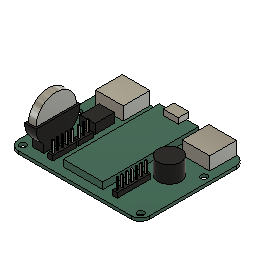
Main_PCB (Autodesk Fusion 360 design; units mm, degrees)
Autodesk Fusion 360 part; units mm, degrees
note: some values were not read from the file. Set by a fixed rule: which sketch regions a step uses.
(part 1 of 3)
sketch "Sketch1" plane through (0, 0, 0) normal (0, 1, 0) x (1, 0, 0)
  line L0 (20.2962, -41.7031) -> (20.1819, -41.6079)
  line L1 (20.1819, -41.6079) -> (20.0105, -41.6079)
  line L2 (20.0105, -41.6079) -> (19.839, -41.7031)
  line L3 (19.839, -41.7031) -> (19.7247, -41.8936)
  line L4 (19.7247, -41.8936) -> (19.6676, -42.0841)
  line L5 (19.6676, -42.0841) -> (19.6105, -42.465)
  line L6 (19.6105, -42.465) -> (19.6105, -42.7507)
  line L7 (19.6105, -42.7507) -> (19.6676, -43.1317)
  line L8 (19.6676, -43.1317) -> (19.7247, -43.3222)
  line L9 (19.7247, -43.3222) -> (19.839, -43.5127)
  line L10 (19.839, -43.5127) -> (20.0105, -43.6079)
  line L11 (20.0105, -43.6079) -> (20.1247, -43.6079)
  line L12 (20.1247, -43.6079) -> (20.2962, -43.5127)
  line L13 (20.2962, -43.5127) -> (20.3533, -43.4174)
  line L14 (20.3533, -43.4174) -> (20.3533, -42.7507)
  line L15 (20.3533, -42.7507) -> (20.1247, -42.7507)
  line L16 (20.8676, -43.6079) -> (20.8676, -41.6079)
  line L17 (20.8676, -41.6079) -> (21.5533, -43.6079)
  line L18 (21.5533, -43.6079) -> (21.5533, -41.6079)
  line L19 (22.1247, -43.6079) -> (22.1247, -41.6079)
  line L20 (22.1247, -41.6079) -> (22.4105, -41.6079)
  line L21 (22.4105, -41.6079) -> (22.5819, -41.7031)
  line L22 (22.5819, -41.7031) -> (22.6962, -41.8936)
  line L23 (22.6962, -41.8936) -> (22.7533, -42.0841)
  line L24 (22.7533, -42.0841) -> (22.8105, -42.465)
  line L25 (22.8105, -42.465) -> (22.8105, -42.7507)
  line L26 (22.8105, -42.7507) -> (22.7533, -43.1317)
  line L27 (22.7533, -43.1317) -> (22.6962, -43.3222)
  line L28 (22.6962, -43.3222) -> (22.5819, -43.5127)
  line L29 (22.5819, -43.5127) -> (22.4105, -43.6079)
  line L30 (22.4105, -43.6079) -> (22.1247, -43.6079)
  line L31 (66.9917, -47.6054) -> (67.0393, -47.4625)
  line L32 (67.0393, -47.4625) -> (67.0393, -47.2244)
  line L33 (67.0393, -47.2244) -> (66.9917, -47.1292)
  line L34 (66.9917, -47.1292) -> (66.9441, -47.0816)
  line L35 (66.9441, -47.0816) -> (66.8489, -47.034)
  line L36 (66.8489, -47.034) -> (66.7536, -47.034)
  line L37 (66.7536, -47.034) -> (66.6584, -47.0816)
  line L38 (66.6584, -47.0816) -> (66.6108, -47.1292)
  line L39 (66.6108, -47.1292) -> (66.5632, -47.2244)
  line L40 (66.5632, -47.2244) -> (66.5155, -47.4149)
  line L41 (66.5155, -47.4149) -> (66.4679, -47.5102)
  line L42 (66.4679, -47.5102) -> (66.4203, -47.5578)
  line L43 (66.4203, -47.5578) -> (66.3251, -47.6054)
  line L44 (66.3251, -47.6054) -> (66.2298, -47.6054)
  line L45 (66.2298, -47.6054) -> (66.1346, -47.5578)
  line L46 (66.1346, -47.5578) -> (66.087, -47.5102)
  line L47 (66.087, -47.5102) -> (66.0393, -47.4149)
  line L48 (66.0393, -47.4149) -> (66.0393, -47.1768)
  line L49 (66.0393, -47.1768) -> (66.087, -47.034)
  line L50 (66.3727, -46.1768) -> (67.0393, -46.1768)
  line L51 (66.3727, -46.6054) -> (66.8965, -46.6054)
  line L52 (66.8965, -46.6054) -> (66.9917, -46.5578)
  line L53 (66.9917, -46.5578) -> (67.0393, -46.4625)
  line L54 (67.0393, -46.4625) -> (67.0393, -46.3197)
  line L55 (67.0393, -46.3197) -> (66.9917, -46.2244)
  line L56 (66.9917, -46.2244) -> (66.9441, -46.1768)
  line L57 (66.3727, -45.7006) -> (67.0393, -45.7006)
  line L58 (66.4679, -45.7006) -> (66.4203, -45.653)
  line L59 (66.4203, -45.653) -> (66.3727, -45.5578)
  line L60 (66.3727, -45.5578) -> (66.3727, -45.4149)
  line L61 (66.3727, -45.4149) -> (66.4203, -45.3197)
  line L62 (66.4203, -45.3197) -> (66.5155, -45.2721)
  line L63 (66.5155, -45.2721) -> (67.0393, -45.2721)
  line L64 (67.0393, -44.7959) -> (66.3727, -44.7959)
  line L65 (66.5632, -44.7959) -> (66.4679, -44.7482)
  line L66 (66.4679, -44.7482) -> (66.4203, -44.7006)
  line L67 (66.4203, -44.7006) -> (66.3727, -44.6054)
  line L68 (66.3727, -44.6054) -> (66.3727, -44.5102)
  line L69 (67.0393, -44.1768) -> (66.3727, -44.1768)
  line L70 (66.0393, -44.1768) -> (66.087, -44.2244)
  line L71 (66.087, -44.2244) -> (66.1346, -44.1768)
  line L72 (66.1346, -44.1768) -> (66.087, -44.1292)
  line L73 (66.087, -44.1292) -> (66.0393, -44.1768)
  line L74 (66.0393, -44.1768) -> (66.1346, -44.1768)
  line L75 (66.9917, -43.7482) -> (67.0393, -43.653)
  line L76 (67.0393, -43.653) -> (67.0393, -43.4625)
  line L77 (67.0393, -43.4625) -> (66.9917, -43.3673)
  line L78 (66.9917, -43.3673) -> (66.8965, -43.3197)
  line L79 (66.8965, -43.3197) -> (66.8489, -43.3197)
  line L80 (66.8489, -43.3197) -> (66.7536, -43.3673)
  line L81 (66.7536, -43.3673) -> (66.706, -43.4625)
  line L82 (66.706, -43.4625) -> (66.706, -43.6054)
  line L83 (66.706, -43.6054) -> (66.6584, -43.7006)
  line L84 (66.6584, -43.7006) -> (66.5632, -43.7482)
  line L85 (66.5632, -43.7482) -> (66.5155, -43.7482)
  line L86 (66.5155, -43.7482) -> (66.4203, -43.7006)
  line L87 (66.4203, -43.7006) -> (66.3727, -43.6054)
  line L88 (66.3727, -43.6054) -> (66.3727, -43.4625)
  line L89 (66.3727, -43.4625) -> (66.4203, -43.3673)
  line L90 (66.9917, -42.5102) -> (67.0393, -42.6054)
  line L91 (67.0393, -42.6054) -> (67.0393, -42.7959)
  line L92 (67.0393, -42.7959) -> (66.9917, -42.8911)
  line L93 (66.9917, -42.8911) -> (66.8965, -42.9387)
  line L94 (66.8965, -42.9387) -> (66.5155, -42.9387)
  line L95 (66.5155, -42.9387) -> (66.4203, -42.8911)
  line L96 (66.4203, -42.8911) -> (66.3727, -42.7959)
  line L97 (66.3727, -42.7959) -> (66.3727, -42.6054)
  line L98 (66.3727, -42.6054) -> (66.4203, -42.5102)
  line L99 (66.4203, -42.5102) -> (66.5155, -42.4625)
  line L100 (66.5155, -42.4625) -> (66.6108, -42.4625)
  line L101 (66.6108, -42.4625) -> (66.706, -42.9387)
  line L102 (66.7536, -41.3197) -> (66.7536, -40.8435)
  line L103 (67.0393, -41.4149) -> (66.0393, -41.0816)
  line L104 (66.0393, -41.0816) -> (67.0393, -40.7482)
  line L105 (67.0393, -40.2721) -> (66.9917, -40.3673)
  line L106 (66.9917, -40.3673) -> (66.8965, -40.4149)
  line L107 (66.8965, -40.4149) -> (66.0393, -40.4149)
  line L108 (67.0393, -39.4625) -> (66.5155, -39.4625)
  line L109 (66.5155, -39.4625) -> (66.4203, -39.5102)
  line L110 (66.4203, -39.5102) -> (66.3727, -39.6054)
  line L111 (66.3727, -39.6054) -> (66.3727, -39.7959)
  line L112 (66.3727, -39.7959) -> (66.4203, -39.8911)
  line L113 (66.9917, -39.4625) -> (67.0393, -39.5578)
  line L114 (67.0393, -39.5578) -> (67.0393, -39.7959)
  line L115 (67.0393, -39.7959) -> (66.9917, -39.8911)
  line L116 (66.9917, -39.8911) -> (66.8965, -39.9387)
  line L117 (66.8965, -39.9387) -> (66.8012, -39.9387)
  line L118 (66.8012, -39.9387) -> (66.706, -39.8911)
  line L119 (66.706, -39.8911) -> (66.6584, -39.7959)
  line L120 (66.6584, -39.7959) -> (66.6584, -39.5578)
  line L121 (66.6584, -39.5578) -> (66.6108, -39.4625)
  line L122 (67.0393, -38.9863) -> (66.3727, -38.9863)
  line L123 (66.5632, -38.9863) -> (66.4679, -38.9387)
  line L124 (66.4679, -38.9387) -> (66.4203, -38.8911)
  line L125 (66.4203, -38.8911) -> (66.3727, -38.7959)
  line L126 (66.3727, -38.7959) -> (66.3727, -38.7006)
  line L127 (67.0393, -38.3673) -> (66.3727, -38.3673)
  line L128 (66.4679, -38.3673) -> (66.4203, -38.3197)
  line L129 (66.4203, -38.3197) -> (66.3727, -38.2244)
  line L130 (66.3727, -38.2244) -> (66.3727, -38.0816)
  line L131 (66.3727, -38.0816) -> (66.4203, -37.9863)
  line L132 (66.4203, -37.9863) -> (66.5155, -37.9387)
  line L133 (66.5155, -37.9387) -> (67.0393, -37.9387)
  line L134 (66.5155, -37.9387) -> (66.4203, -37.8911)
  line L135 (66.4203, -37.8911) -> (66.3727, -37.7959)
  line L136 (66.3727, -37.7959) -> (66.3727, -37.653)
  line L137 (66.3727, -37.653) -> (66.4203, -37.5578)
  line L138 (66.4203, -37.5578) -> (66.5155, -37.5102)
  line L139 (66.5155, -37.5102) -> (67.0393, -37.5102)
  line L140 (66.0393, -36.4149) -> (67.0393, -36.0816)
  line L141 (67.0393, -36.0816) -> (66.0393, -35.7482)
  line L142 (66.0393, -35.5102) -> (66.0393, -34.8911)
  line L143 (66.0393, -34.8911) -> (66.4203, -35.2244)
  line L144 (66.4203, -35.2244) -> (66.4203, -35.0816)
  line L145 (66.4203, -35.0816) -> (66.4679, -34.9863)
  line L146 (66.4679, -34.9863) -> (66.5155, -34.9387)
  line L147 (66.5155, -34.9387) -> (66.6108, -34.8911)
  line L148 (66.6108, -34.8911) -> (66.8489, -34.8911)
  line L149 (66.8489, -34.8911) -> (66.9441, -34.9387)
  line L150 (66.9441, -34.9387) -> (66.9917, -34.9863)
  line L151 (66.9917, -34.9863) -> (67.0393, -35.0816)
  line L152 (67.0393, -35.0816) -> (67.0393, -35.3673)
  line L153 (67.0393, -35.3673) -> (66.9917, -35.4625)
  line L154 (66.9917, -35.4625) -> (66.9441, -35.5102)
  line L155 (66.9441, -34.4625) -> (66.9917, -34.4149)
  line L156 (66.9917, -34.4149) -> (67.0393, -34.4625)
  line L157 (67.0393, -34.4625) -> (66.9917, -34.5102)
  line L158 (66.9917, -34.5102) -> (66.9441, -34.4625)
  line L159 (66.9441, -34.4625) -> (67.0393, -34.4625)
  line L160 (66.4203, -34.4625) -> (66.4679, -34.4149)
  line L161 (66.4679, -34.4149) -> (66.5155, -34.4625)
  line L162 (66.5155, -34.4625) -> (66.4679, -34.5102)
  line L163 (66.4679, -34.5102) -> (66.4203, -34.4625)
  line L164 (66.4203, -34.4625) -> (66.5155, -34.4625)
  line L165 (67.0393, -33.2244) -> (66.0393, -33.2244)
  line L166 (66.0393, -33.2244) -> (66.7536, -32.8911)
  line L167 (66.7536, -32.8911) -> (66.0393, -32.5578)
  line L168 (66.0393, -32.5578) -> (67.0393, -32.5578)
  line L169 (67.0393, -31.653) -> (66.5155, -31.653)
  line L170 (66.5155, -31.653) -> (66.4203, -31.7006)
  line L171 (66.4203, -31.7006) -> (66.3727, -31.7959)
  line L172 (66.3727, -31.7959) -> (66.3727, -31.9863)
  line L173 (66.3727, -31.9863) -> (66.4203, -32.0816)
  line L174 (66.9917, -31.653) -> (67.0393, -31.7482)
  line L175 (67.0393, -31.7482) -> (67.0393, -31.9863)
  line L176 (67.0393, -31.9863) -> (66.9917, -32.0816)
  line L177 (66.9917, -32.0816) -> (66.8965, -32.1292)
  line L178 (66.8965, -32.1292) -> (66.8012, -32.1292)
  line L179 (66.8012, -32.1292) -> (66.706, -32.0816)
  line L180 (66.706, -32.0816) -> (66.6584, -31.9863)
  line L181 (66.6584, -31.9863) -> (66.6584, -31.7482)
  line L182 (66.6584, -31.7482) -> (66.6108, -31.653)
  line L183 (67.0393, -31.1768) -> (66.3727, -31.1768)
  line L184 (66.0393, -31.1768) -> (66.087, -31.2244)
  line L185 (66.087, -31.2244) -> (66.1346, -31.1768)
  line L186 (66.1346, -31.1768) -> (66.087, -31.1292)
  line L187 (66.087, -31.1292) -> (66.0393, -31.1768)
  line L188 (66.0393, -31.1768) -> (66.1346, -31.1768)
  line L189 (66.3727, -30.7006) -> (67.0393, -30.7006)
  line L190 (66.4679, -30.7006) -> (66.4203, -30.653)
  line L191 (66.4203, -30.653) -> (66.3727, -30.5578)
  line L192 (66.3727, -30.5578) -> (66.3727, -30.4149)
  line L193 (66.3727, -30.4149) -> (66.4203, -30.3197)
  line L194 (66.4203, -30.3197) -> (66.5155, -30.2721)
  line L195 (66.5155, -30.2721) -> (67.0393, -30.2721)
  line L196 (67.0393, -29.034) -> (66.0393, -29.034)
  line L197 (66.0393, -29.034) -> (66.0393, -28.653)
  line L198 (66.0393, -28.653) -> (66.087, -28.5578)
  line L199 (66.087, -28.5578) -> (66.1346, -28.5102)
  line L200 (66.1346, -28.5102) -> (66.2298, -28.4625)
  line L201 (66.2298, -28.4625) -> (66.3727, -28.4625)
  line L202 (66.3727, -28.4625) -> (66.4679, -28.5102)
  line L203 (66.4679, -28.5102) -> (66.5155, -28.5578)
  line L204 (66.5155, -28.5578) -> (66.5632, -28.653)
  line L205 (66.5632, -28.653) -> (66.5632, -29.034)
  line L206 (66.9441, -27.4625) -> (66.9917, -27.5102)
  line L207 (66.9917, -27.5102) -> (67.0393, -27.653)
  line L208 (67.0393, -27.653) -> (67.0393, -27.7482)
  line L209 (67.0393, -27.7482) -> (66.9917, -27.8911)
  line L210 (66.9917, -27.8911) -> (66.8965, -27.9863)
  line L211 (66.8965, -27.9863) -> (66.8012, -28.034)
  line L212 (66.8012, -28.034) -> (66.6108, -28.0816)
  line L213 (66.6108, -28.0816) -> (66.4679, -28.0816)
  line L214 (66.4679, -28.0816) -> (66.2774, -28.034)
  line L215 (66.2774, -28.034) -> (66.1822, -27.9863)
  line L216 (66.1822, -27.9863) -> (66.087, -27.8911)
  line L217 (66.087, -27.8911) -> (66.0393, -27.7482)
  line L218 (66.0393, -27.7482) -> (66.0393, -27.653)
  line L219 (66.0393, -27.653) -> (66.087, -27.5102)
  line L220 (66.087, -27.5102) -> (66.1346, -27.4625)
  line L221 (66.5155, -26.7006) -> (66.5632, -26.5578)
  line L222 (66.5632, -26.5578) -> (66.6108, -26.5102)
  line L223 (66.6108, -26.5102) -> (66.706, -26.4625)
  line L224 (66.706, -26.4625) -> (66.8489, -26.4625)
  line L225 (66.8489, -26.4625) -> (66.9441, -26.5102)
  line L226 (66.9441, -26.5102) -> (66.9917, -26.5578)
  line L227 (66.9917, -26.5578) -> (67.0393, -26.653)
  line L228 (67.0393, -26.653) -> (67.0393, -27.034)
  line L229 (67.0393, -27.034) -> (66.0393, -27.034)
  line L230 (66.0393, -27.034) -> (66.0393, -26.7006)
  line L231 (66.0393, -26.7006) -> (66.087, -26.6054)
  line L232 (66.087, -26.6054) -> (66.1346, -26.5578)
  line L233 (66.1346, -26.5578) -> (66.2298, -26.5102)
  line L234 (66.2298, -26.5102) -> (66.3251, -26.5102)
  line L235 (66.3251, -26.5102) -> (66.4203, -26.5578)
  line L236 (66.4203, -26.5578) -> (66.4679, -26.6054)
  line L237 (66.4679, -26.6054) -> (66.5155, -26.7006)
  line L238 (66.5155, -26.7006) -> (66.5155, -27.034)
  line L239 (66.0393, -25.4149) -> (67.0393, -25.0816)
  line L240 (67.0393, -25.0816) -> (66.0393, -24.7482)
  line L241 (67.0393, -23.8911) -> (67.0393, -24.4625)
  line L242 (67.0393, -24.1768) -> (66.0393, -24.1768)
  line L243 (66.0393, -24.1768) -> (66.1822, -24.2721)
  line L244 (66.1822, -24.2721) -> (66.2774, -24.3673)
  line L245 (66.2774, -24.3673) -> (66.3251, -24.4625)
  line L246 (19.8962, -35.4079) -> (20.1247, -35.4079)
  line L247 (20.1247, -35.4079) -> (20.239, -35.5031)
  line L248 (20.239, -35.5031) -> (20.3533, -35.6936)
  line L249 (20.3533, -35.6936) -> (20.4105, -36.0746)
  line L250 (20.4105, -36.0746) -> (20.4105, -36.7412)
  line L251 (20.4105, -36.7412) -> (20.3533, -37.1222)
  line L252 (20.3533, -37.1222) -> (20.239, -37.3126)
  line L253 (20.239, -37.3126) -> (20.1247, -37.4079)
  line L254 (20.1247, -37.4079) -> (19.8962, -37.4079)
  line L255 (19.8962, -37.4079) -> (19.7819, -37.3126)
  line L256 (19.7819, -37.3126) -> (19.6676, -37.1222)
  line L257 (19.6676, -37.1222) -> (19.6105, -36.7412)
  line L258 (19.6105, -36.7412) -> (19.6105, -36.0746)
  line L259 (19.6105, -36.0746) -> (19.6676, -35.6936)
  line L260 (19.6676, -35.6936) -> (19.7819, -35.5031)
  line L261 (19.7819, -35.5031) -> (19.8962, -35.4079)
  line L262 (20.9247, -35.4079) -> (20.9247, -37.0269)
  line L263 (20.9247, -37.0269) -> (20.9819, -37.2174)
  line L264 (20.9819, -37.2174) -> (21.039, -37.3126)
  line L265 (21.039, -37.3126) -> (21.1533, -37.4079)
  line L266 (21.1533, -37.4079) -> (21.3819, -37.4079)
  line L267 (21.3819, -37.4079) -> (21.4962, -37.3126)
  line L268 (21.4962, -37.3126) -> (21.5533, -37.2174)
  line L269 (21.5533, -37.2174) -> (21.6105, -37.0269)
  line L270 (21.6105, -37.0269) -> (21.6105, -35.4079)
  line L271 (22.0105, -35.4079) -> (22.6962, -35.4079)
  line L272 (22.3533, -37.4079) -> (22.3533, -35.4079)
  line L273 (20.3533, -46.1079) -> (19.9533, -45.1555)
  line L274 (19.6676, -46.1079) -> (19.6676, -44.1079)
  line L275 (19.6676, -44.1079) -> (20.1247, -44.1079)
  line L276 (20.1247, -44.1079) -> (20.239, -44.2031)
  line L277 (20.239, -44.2031) -> (20.2962, -44.2984)
  line L278 (20.2962, -44.2984) -> (20.3533, -44.4888)
  line L279 (20.3533, -44.4888) -> (20.3533, -44.7746)
  line L280 (20.3533, -44.7746) -> (20.2962, -44.965)
  line L281 (20.2962, -44.965) -> (20.239, -45.0603)
  line L282 (20.239, -45.0603) -> (20.1247, -45.1555)
  line L283 (20.1247, -45.1555) -> (19.6676, -45.1555)
  line L284 (20.8676, -46.1079) -> (20.8676, -44.1079)
  line L285 (22.0676, -44.2031) -> (21.9533, -44.1079)
  line L286 (21.9533, -44.1079) -> (21.7819, -44.1079)
  line L287 (21.7819, -44.1079) -> (21.6105, -44.2031)
  line L288 (21.6105, -44.2031) -> (21.4962, -44.3936)
  line L289 (21.4962, -44.3936) -> (21.439, -44.5841)
  line L290 (21.439, -44.5841) -> (21.3819, -44.965)
  line L291 (21.3819, -44.965) -> (21.3819, -45.2507)
  line L292 (21.3819, -45.2507) -> (21.439, -45.6317)
  line L293 (21.439, -45.6317) -> (21.4962, -45.8222)
  line L294 (21.4962, -45.8222) -> (21.6105, -46.0127)
  line L295 (21.6105, -46.0127) -> (21.7819, -46.1079)
  line L296 (21.7819, -46.1079) -> (21.8962, -46.1079)
  line L297 (21.8962, -46.1079) -> (22.0676, -46.0127)
  line L298 (22.0676, -46.0127) -> (22.1247, -45.9174)
  line L299 (22.1247, -45.9174) -> (22.1247, -45.2507)
  line L300 (22.1247, -45.2507) -> (21.8962, -45.2507)
  line L301 (48.1872, -43.3174) -> (48.13, -43.4126)
  line L302 (48.13, -43.4126) -> (47.9586, -43.5079)
  line L303 (47.9586, -43.5079) -> (47.8443, -43.5079)
  line L304 (47.8443, -43.5079) -> (47.6729, -43.4126)
  line L305 (47.6729, -43.4126) -> (47.5586, -43.2222)
  line L306 (47.5586, -43.2222) -> (47.5014, -43.0317)
  line L307 (47.5014, -43.0317) -> (47.4443, -42.6507)
  line L308 (47.4443, -42.6507) -> (47.4443, -42.365)
  line L309 (47.4443, -42.365) -> (47.5014, -41.9841)
  line L310 (47.5014, -41.9841) -> (47.5586, -41.7936)
  line L311 (47.5586, -41.7936) -> (47.6729, -41.6031)
  line L312 (47.6729, -41.6031) -> (47.8443, -41.5079)
  line L313 (47.8443, -41.5079) -> (47.9586, -41.5079)
  line L314 (47.9586, -41.5079) -> (48.13, -41.6031)
  line L315 (48.13, -41.6031) -> (48.1872, -41.6984)
  line L316 (49.2729, -43.5079) -> (48.7014, -43.5079)
  line L317 (48.7014, -43.5079) -> (48.7014, -41.5079)
  line L318 (49.6729, -43.5079) -> (49.6729, -41.5079)
  line L319 (50.3586, -43.5079) -> (49.8443, -42.365)
  line L320 (50.3586, -41.5079) -> (49.6729, -42.6507)
  line L321 (48.4729, -48.6079) -> (48.4729, -46.6079)
  line L322 (48.4729, -46.6079) -> (48.7586, -46.6079)
  line L323 (48.7586, -46.6079) -> (48.93, -46.7031)
  line L324 (48.93, -46.7031) -> (49.0443, -46.8936)
  line L325 (49.0443, -46.8936) -> (49.1014, -47.0841)
  line L326 (49.1014, -47.0841) -> (49.1586, -47.465)
  line L327 (49.1586, -47.465) -> (49.1586, -47.7507)
  line L328 (49.1586, -47.7507) -> (49.1014, -48.1317)
  line L329 (49.1014, -48.1317) -> (49.0443, -48.3222)
  line L330 (49.0443, -48.3222) -> (48.93, -48.5127)
  line L331 (48.93, -48.5127) -> (48.7586, -48.6079)
  line L332 (48.7586, -48.6079) -> (48.4729, -48.6079)
  line L333 (50.3586, -48.4174) -> (50.3014, -48.5127)
  line L334 (50.3014, -48.5127) -> (50.13, -48.6079)
  line L335 (50.13, -48.6079) -> (50.0157, -48.6079)
  line L336 (50.0157, -48.6079) -> (49.8443, -48.5127)
  line L337 (49.8443, -48.5127) -> (49.73, -48.3222)
  line L338 (49.73, -48.3222) -> (49.6729, -48.1317)
  line L339 (49.6729, -48.1317) -> (49.6157, -47.7507)
  line L340 (49.6157, -47.7507) -> (49.6157, -47.465)
  line L341 (49.6157, -47.465) -> (49.6729, -47.0841)
  line L342 (49.6729, -47.0841) -> (49.73, -46.8936)
  line L343 (49.73, -46.8936) -> (49.8443, -46.7031)
  line L344 (49.8443, -46.7031) -> (50.0157, -46.6079)
  line L345 (50.0157, -46.6079) -> (50.13, -46.6079)
  line L346 (50.13, -46.6079) -> (50.3014, -46.7031)
  line L347 (50.3014, -46.7031) -> (50.3586, -46.7984)
  line L348 (48.3014, -51.2079) -> (47.9014, -50.2555)
  line L349 (47.6157, -51.2079) -> (47.6157, -49.2079)
  line L350 (47.6157, -49.2079) -> (48.0729, -49.2079)
  line L351 (48.0729, -49.2079) -> (48.1872, -49.3031)
  line L352 (48.1872, -49.3031) -> (48.2443, -49.3984)
  line L353 (48.2443, -49.3984) -> (48.3014, -49.5888)
  line L354 (48.3014, -49.5888) -> (48.3014, -49.8746)
  line L355 (48.3014, -49.8746) -> (48.2443, -50.065)
  line L356 (48.2443, -50.065) -> (48.1872, -50.1603)
  line L357 (48.1872, -50.1603) -> (48.0729, -50.2555)
  line L358 (48.0729, -50.2555) -> (47.6157, -50.2555)
  line L359 (48.7586, -51.1126) -> (48.93, -51.2079)
  line L360 (48.93, -51.2079) -> (49.2157, -51.2079)
  line L361 (49.2157, -51.2079) -> (49.33, -51.1126)
  line L362 (49.33, -51.1126) -> (49.3872, -51.0174)
  line L363 (49.3872, -51.0174) -> (49.4443, -50.8269)
  line L364 (49.4443, -50.8269) -> (49.4443, -50.6365)
  line L365 (49.4443, -50.6365) -> (49.3872, -50.446)
  line L366 (49.3872, -50.446) -> (49.33, -50.3507)
  line L367 (49.33, -50.3507) -> (49.2157, -50.2555)
  line L368 (49.2157, -50.2555) -> (48.9872, -50.1603)
  line L369 (48.9872, -50.1603) -> (48.8729, -50.065)
  line L370 (48.8729, -50.065) -> (48.8157, -49.9698)
  line L371 (48.8157, -49.9698) -> (48.7586, -49.7793)
  line L372 (48.7586, -49.7793) -> (48.7586, -49.5888)
  line L373 (48.7586, -49.5888) -> (48.8157, -49.3984)
  line L374 (48.8157, -49.3984) -> (48.8729, -49.3031)
  line L375 (48.8729, -49.3031) -> (48.9872, -49.2079)
  line L376 (48.9872, -49.2079) -> (49.2729, -49.2079)
  line L377 (49.2729, -49.2079) -> (49.4443, -49.3031)
  line L378 (49.7872, -49.2079) -> (50.4729, -49.2079)
  line L379 (50.13, -51.2079) -> (50.13, -49.2079)
  line L380 (20.239, -51.3079) -> (19.6676, -51.3079)
  line L381 (19.6676, -51.3079) -> (19.6676, -49.3079)
  line L382 (20.639, -50.2603) -> (21.039, -50.2603)
  line L383 (21.2105, -51.3079) -> (20.639, -51.3079)
  line L384 (20.639, -51.3079) -> (20.639, -49.3079)
  line L385 (20.639, -49.3079) -> (21.2105, -49.3079)
  line L386 (22.1247, -50.2603) -> (21.7247, -50.2603)
  line L387 (21.7247, -51.3079) -> (21.7247, -49.3079)
  line L388 (21.7247, -49.3079) -> (22.2962, -49.3079)
  line L389 (49.2157, -45.9174) -> (49.1586, -46.0127)
  line L390 (49.1586, -46.0127) -> (48.9872, -46.1079)
  line L391 (48.9872, -46.1079) -> (48.8729, -46.1079)
  line L392 (48.8729, -46.1079) -> (48.7014, -46.0127)
  line L393 (48.7014, -46.0127) -> (48.5872, -45.8222)
  line L394 (48.5872, -45.8222) -> (48.53, -45.6317)
  line L395 (48.53, -45.6317) -> (48.4729, -45.2507)
  line L396 (48.4729, -45.2507) -> (48.4729, -44.965)
  line L397 (48.4729, -44.965) -> (48.53, -44.5841)
  line L398 (48.53, -44.5841) -> (48.5872, -44.3936)
  line L399 (48.5872, -44.3936) -> (48.7014, -44.2031)
  line L400 (48.7014, -44.2031) -> (48.8729, -44.1079)
  line L401 (48.8729, -44.1079) -> (48.9872, -44.1079)
  line L402 (48.9872, -44.1079) -> (49.1586, -44.2031)
  line L403 (49.1586, -44.2031) -> (49.2157, -44.2984)
  line L404 (49.6729, -46.0127) -> (49.8443, -46.1079)
  line L405 (49.8443, -46.1079) -> (50.13, -46.1079)
  line L406 (50.13, -46.1079) -> (50.2443, -46.0127)
  line L407 (50.2443, -46.0127) -> (50.3014, -45.9174)
  line L408 (50.3014, -45.9174) -> (50.3586, -45.7269)
  line L409 (50.3586, -45.7269) -> (50.3586, -45.5365)
  line L410 (50.3586, -45.5365) -> (50.3014, -45.346)
  line L411 (50.3014, -45.346) -> (50.2443, -45.2507)
  line L412 (50.2443, -45.2507) -> (50.13, -45.1555)
  line L413 (50.13, -45.1555) -> (49.9014, -45.0603)
  line L414 (49.9014, -45.0603) -> (49.7872, -44.965)
  line L415 (49.7872, -44.965) -> (49.73, -44.8698)
  line L416 (49.73, -44.8698) -> (49.6729, -44.6793)
  line L417 (49.6729, -44.6793) -> (49.6729, -44.4888)
  line L418 (49.6729, -44.4888) -> (49.73, -44.2984)
  line L419 (49.73, -44.2984) -> (49.7872, -44.2031)
  line L420 (49.7872, -44.2031) -> (49.9014, -44.1079)
  line L421 (49.9014, -44.1079) -> (50.1872, -44.1079)
  line L422 (50.1872, -44.1079) -> (50.3586, -44.2031)
  line L423 (20.2962, -33.0031) -> (20.1819, -32.9079)
  line L424 (20.1819, -32.9079) -> (20.0105, -32.9079)
  line L425 (20.0105, -32.9079) -> (19.839, -33.0031)
  line L426 (19.839, -33.0031) -> (19.7247, -33.1936)
  line L427 (19.7247, -33.1936) -> (19.6676, -33.3841)
  line L428 (19.6676, -33.3841) -> (19.6105, -33.765)
  line L429 (19.6105, -33.765) -> (19.6105, -34.0507)
  line L430 (19.6105, -34.0507) -> (19.6676, -34.4317)
  line L431 (19.6676, -34.4317) -> (19.7247, -34.6222)
  line L432 (19.7247, -34.6222) -> (19.839, -34.8126)
  line L433 (19.839, -34.8126) -> (20.0105, -34.9079)
  line L434 (20.0105, -34.9079) -> (20.1247, -34.9079)
  line L435 (20.1247, -34.9079) -> (20.2962, -34.8126)
  line L436 (20.2962, -34.8126) -> (20.3533, -34.7174)
  line L437 (20.3533, -34.7174) -> (20.3533, -34.0507)
  line L438 (20.3533, -34.0507) -> (20.1247, -34.0507)
  line L439 (20.8676, -34.9079) -> (20.8676, -32.9079)
  line L440 (20.8676, -32.9079) -> (21.5533, -34.9079)
  line L441 (21.5533, -34.9079) -> (21.5533, -32.9079)
  line L442 (22.1247, -34.9079) -> (22.1247, -32.9079)
  line L443 (22.1247, -32.9079) -> (22.4105, -32.9079)
  line L444 (22.4105, -32.9079) -> (22.5819, -33.0031)
  line L445 (22.5819, -33.0031) -> (22.6962, -33.1936)
  line L446 (22.6962, -33.1936) -> (22.7533, -33.3841)
  line L447 (22.7533, -33.3841) -> (22.8105, -33.765)
  line L448 (22.8105, -33.765) -> (22.8105, -34.0507)
  line L449 (22.8105, -34.0507) -> (22.7533, -34.4317)
  line L450 (22.7533, -34.4317) -> (22.6962, -34.6222)
  line L451 (22.6962, -34.6222) -> (22.5819, -34.8126)
  line L452 (22.5819, -34.8126) -> (22.4105, -34.9079)
  line L453 (22.4105, -34.9079) -> (22.1247, -34.9079)
  line L454 (47.8443, -41.0079) -> (47.8443, -39.0079)
  line L455 (47.8443, -39.0079) -> (48.13, -39.0079)
  line L456 (48.13, -39.0079) -> (48.3014, -39.1031)
  line L457 (48.3014, -39.1031) -> (48.4157, -39.2936)
  line L458 (48.4157, -39.2936) -> (48.4729, -39.4841)
  line L459 (48.4729, -39.4841) -> (48.53, -39.865)
  line L460 (48.53, -39.865) -> (48.53, -40.1507)
  line L461 (48.53, -40.1507) -> (48.4729, -40.5317)
  line L462 (48.4729, -40.5317) -> (48.4157, -40.7222)
  line L463 (48.4157, -40.7222) -> (48.3014, -40.9126)
  line L464 (48.3014, -40.9126) -> (48.13, -41.0079)
  line L465 (48.13, -41.0079) -> (47.8443, -41.0079)
  line L466 (49.0443, -41.0079) -> (49.0443, -39.0079)
  line L467 (49.6157, -41.0079) -> (49.6157, -39.0079)
  line L468 (49.6157, -39.0079) -> (50.3014, -41.0079)
  line L469 (50.3014, -41.0079) -> (50.3014, -39.0079)
  line L470 (19.4362, -30.4079) -> (19.8362, -32.4079)
  line L471 (19.8362, -32.4079) -> (20.2362, -30.4079)
  line L472 (21.3219, -32.2174) -> (21.2647, -32.3126)
  line L473 (21.2647, -32.3126) -> (21.0933, -32.4079)
  line L474 (21.0933, -32.4079) -> (20.979, -32.4079)
  line L475 (20.979, -32.4079) -> (20.8076, -32.3126)
  line L476 (20.8076, -32.3126) -> (20.6933, -32.1222)
  line L477 (20.6933, -32.1222) -> (20.6362, -31.9317)
  line L478 (20.6362, -31.9317) -> (20.579, -31.5507)
  line L479 (20.579, -31.5507) -> (20.579, -31.265)
  line L480 (20.579, -31.265) -> (20.6362, -30.8841)
  line L481 (20.6362, -30.8841) -> (20.6933, -30.6936)
  line L482 (20.6933, -30.6936) -> (20.8076, -30.5031)
  line L483 (20.8076, -30.5031) -> (20.979, -30.4079)
  line L484 (20.979, -30.4079) -> (21.0933, -30.4079)
  line L485 (21.0933, -30.4079) -> (21.2647, -30.5031)
  line L486 (21.2647, -30.5031) -> (21.3219, -30.5984)
  line L487 (22.5219, -32.2174) -> (22.4647, -32.3126)
  line L488 (22.4647, -32.3126) -> (22.2933, -32.4079)
  line L489 (22.2933, -32.4079) -> (22.179, -32.4079)
  line L490 (22.179, -32.4079) -> (22.0076, -32.3126)
  line L491 (22.0076, -32.3126) -> (21.8933, -32.1222)
  line L492 (21.8933, -32.1222) -> (21.8362, -31.9317)
  line L493 (21.8362, -31.9317) -> (21.779, -31.5507)
  line L494 (21.779, -31.5507) -> (21.779, -31.265)
  line L495 (21.779, -31.265) -> (21.8362, -30.8841)
  line L496 (21.8362, -30.8841) -> (21.8933, -30.6936)
  line L497 (21.8933, -30.6936) -> (22.0076, -30.5031)
  line L498 (22.0076, -30.5031) -> (22.179, -30.4079)
  line L499 (22.179, -30.4079) -> (22.2933, -30.4079)
  line L500 (22.2933, -30.4079) -> (22.4647, -30.5031)
  line L501 (22.4647, -30.5031) -> (22.5219, -30.5984)
  line L502 (47.8343, -36.6031) -> (47.72, -36.5079)
  line L503 (47.72, -36.5079) -> (47.5486, -36.5079)
  line L504 (47.5486, -36.5079) -> (47.3772, -36.6031)
  line L505 (47.3772, -36.6031) -> (47.2629, -36.7936)
  line L506 (47.2629, -36.7936) -> (47.2057, -36.9841)
  line L507 (47.2057, -36.9841) -> (47.1486, -37.365)
  line L508 (47.1486, -37.365) -> (47.1486, -37.6507)
  line L509 (47.1486, -37.6507) -> (47.2057, -38.0317)
  line L510 (47.2057, -38.0317) -> (47.2629, -38.2222)
  line L511 (47.2629, -38.2222) -> (47.3772, -38.4126)
  line L512 (47.3772, -38.4126) -> (47.5486, -38.5079)
  line L513 (47.5486, -38.5079) -> (47.6629, -38.5079)
  line L514 (47.6629, -38.5079) -> (47.8343, -38.4126)
  line L515 (47.8343, -38.4126) -> (47.8914, -38.3174)
  line L516 (47.8914, -38.3174) -> (47.8914, -37.6507)
  line L517 (47.8914, -37.6507) -> (47.6629, -37.6507)
  line L518 (48.4057, -38.5079) -> (48.4057, -36.5079)
  line L519 (48.4057, -36.5079) -> (49.0914, -38.5079)
  line L520 (49.0914, -38.5079) -> (49.0914, -36.5079)
  line L521 (49.6629, -38.5079) -> (49.6629, -36.5079)
  line L522 (49.6629, -36.5079) -> (49.9486, -36.5079)
  line L523 (49.9486, -36.5079) -> (50.12, -36.6031)
  line L524 (50.12, -36.6031) -> (50.2343, -36.7936)
  line L525 (50.2343, -36.7936) -> (50.2914, -36.9841)
  line L526 (50.2914, -36.9841) -> (50.3486, -37.365)
  line L527 (50.3486, -37.365) -> (50.3486, -37.6507)
  line L528 (50.3486, -37.6507) -> (50.2914, -38.0317)
  line L529 (50.2914, -38.0317) -> (50.2343, -38.2222)
  line L530 (50.2343, -38.2222) -> (50.12, -38.4126)
  line L531 (50.12, -38.4126) -> (49.9486, -38.5079)
  line L532 (49.9486, -38.5079) -> (49.6629, -38.5079)
  line L533 (19.4962, -39.1079) -> (19.8962, -41.1079)
  line L534 (19.8962, -41.1079) -> (20.2962, -39.1079)
  line L535 (21.3819, -40.9174) -> (21.3247, -41.0127)
  line L536 (21.3247, -41.0127) -> (21.1533, -41.1079)
  line L537 (21.1533, -41.1079) -> (21.039, -41.1079)
  line L538 (21.039, -41.1079) -> (20.8676, -41.0127)
  line L539 (20.8676, -41.0127) -> (20.7533, -40.8222)
  line L540 (20.7533, -40.8222) -> (20.6962, -40.6317)
  line L541 (20.6962, -40.6317) -> (20.639, -40.2507)
  line L542 (20.639, -40.2507) -> (20.639, -39.965)
  line L543 (20.639, -39.965) -> (20.6962, -39.5841)
  line L544 (20.6962, -39.5841) -> (20.7533, -39.3936)
  line L545 (20.7533, -39.3936) -> (20.8676, -39.2031)
  line L546 (20.8676, -39.2031) -> (21.039, -39.1079)
  line L547 (21.039, -39.1079) -> (21.1533, -39.1079)
  line L548 (21.1533, -39.1079) -> (21.3247, -39.2031)
  line L549 (21.3247, -39.2031) -> (21.3819, -39.2984)
  line L550 (22.5819, -40.9174) -> (22.5247, -41.0127)
  line L551 (22.5247, -41.0127) -> (22.3533, -41.1079)
  line L552 (22.3533, -41.1079) -> (22.239, -41.1079)
  line L553 (22.239, -41.1079) -> (22.0676, -41.0127)
  line L554 (22.0676, -41.0127) -> (21.9533, -40.8222)
  line L555 (21.9533, -40.8222) -> (21.8962, -40.6317)
  line L556 (21.8962, -40.6317) -> (21.839, -40.2507)
  line L557 (21.839, -40.2507) -> (21.839, -39.965)
  line L558 (21.839, -39.965) -> (21.8962, -39.5841)
  line L559 (21.8962, -39.5841) -> (21.9533, -39.3936)
  line L560 (21.9533, -39.3936) -> (22.0676, -39.2031)
  line L561 (22.0676, -39.2031) -> (22.239, -39.1079)
  line L562 (22.239, -39.1079) -> (22.3533, -39.1079)
  line L563 (22.3533, -39.1079) -> (22.5247, -39.2031)
  line L564 (22.5247, -39.2031) -> (22.5819, -39.2984)
  line L565 (19.6676, -48.7079) -> (19.6676, -46.7079)
  line L566 (19.6676, -46.7079) -> (20.0676, -48.1365)
  line L567 (20.0676, -48.1365) -> (20.4676, -46.7079)
  line L568 (20.4676, -46.7079) -> (20.4676, -48.7079)
  line L569 (21.039, -48.7079) -> (21.039, -46.7079)
  line L570 (21.6105, -48.7079) -> (21.6105, -46.7079)
  line L571 (21.6105, -46.7079) -> (21.8962, -46.7079)
  line L572 (21.8962, -46.7079) -> (22.0676, -46.8031)
  line L573 (22.0676, -46.8031) -> (22.1819, -46.9936)
  line L574 (22.1819, -46.9936) -> (22.239, -47.1841)
  line L575 (22.239, -47.1841) -> (22.2962, -47.565)
  line L576 (22.2962, -47.565) -> (22.2962, -47.8507)
  line L577 (22.2962, -47.8507) -> (22.239, -48.2317)
  line L578 (22.239, -48.2317) -> (22.1819, -48.4222)
  line L579 (22.1819, -48.4222) -> (22.0676, -48.6126)
  line L580 (22.0676, -48.6126) -> (21.8962, -48.7079)
  line L581 (21.8962, -48.7079) -> (21.6105, -48.7079)
  line L582 (47.2629, -33.9554) -> (47.6629, -35.9554)
  line L583 (47.6629, -35.9554) -> (48.0629, -33.9554)
  line L584 (49.1486, -35.7649) -> (49.0914, -35.8601)
  line L585 (49.0914, -35.8601) -> (48.92, -35.9554)
  line L586 (48.92, -35.9554) -> (48.8057, -35.9554)
  line L587 (48.8057, -35.9554) -> (48.6343, -35.8601)
  line L588 (48.6343, -35.8601) -> (48.52, -35.6697)
  line L589 (48.52, -35.6697) -> (48.4629, -35.4792)
  line L590 (48.4629, -35.4792) -> (48.4057, -35.0982)
  line L591 (48.4057, -35.0982) -> (48.4057, -34.8125)
  line L592 (48.4057, -34.8125) -> (48.4629, -34.4316)
  line L593 (48.4629, -34.4316) -> (48.52, -34.2411)
  line L594 (48.52, -34.2411) -> (48.6343, -34.0506)
  line L595 (48.6343, -34.0506) -> (48.8057, -33.9554)
  line L596 (48.8057, -33.9554) -> (48.92, -33.9554)
  line L597 (48.92, -33.9554) -> (49.0914, -34.0506)
  line L598 (49.0914, -34.0506) -> (49.1486, -34.1459)
  line L599 (50.3486, -35.7649) -> (50.2914, -35.8601)
  line L600 (50.2914, -35.8601) -> (50.12, -35.9554)
  line L601 (50.12, -35.9554) -> (50.0057, -35.9554)
  line L602 (50.0057, -35.9554) -> (49.8343, -35.8601)
  line L603 (49.8343, -35.8601) -> (49.72, -35.6697)
  line L604 (49.72, -35.6697) -> (49.6629, -35.4792)
  line L605 (49.6629, -35.4792) -> (49.6057, -35.0982)
  line L606 (49.6057, -35.0982) -> (49.6057, -34.8125)
  line L607 (49.6057, -34.8125) -> (49.6629, -34.4316)
  line L608 (49.6629, -34.4316) -> (49.72, -34.2411)
  line L609 (49.72, -34.2411) -> (49.8343, -34.0506)
  line L610 (49.8343, -34.0506) -> (50.0057, -33.9554)
  line L611 (50.0057, -33.9554) -> (50.12, -33.9554)
  line L612 (50.12, -33.9554) -> (50.2914, -34.0506)
  line L613 (50.2914, -34.0506) -> (50.3486, -34.1459)
  line L614 (17.2012, -15.1656) -> (17.2012, -15.8799)
  line L615 (17.2012, -15.8799) -> (17.1536, -16.0227)
  line L616 (17.1536, -16.0227) -> (17.0583, -16.118)
  line L617 (17.0583, -16.118) -> (16.9155, -16.1656)
  line L618 (16.9155, -16.1656) -> (16.8202, -16.1656)
  line L619 (18.106, -15.4989) -> (18.106, -16.1656)
  line L620 (17.8679, -15.118) -> (17.6298, -15.8322)
  line L621 (17.6298, -15.8322) -> (18.2488, -15.8322)
  line L622 (3.0393, -6.9863) -> (3.8489, -6.9863)
  line L623 (3.8489, -6.9863) -> (3.9441, -6.9387)
  line L624 (3.9441, -6.9387) -> (3.9917, -6.8911)
  line L625 (3.9917, -6.8911) -> (4.0393, -6.7959)
  line L626 (4.0393, -6.7959) -> (4.0393, -6.6054)
  line L627 (4.0393, -6.6054) -> (3.9917, -6.5102)
  line L628 (3.9917, -6.5102) -> (3.9441, -6.4625)
  line L629 (3.9441, -6.4625) -> (3.8489, -6.4149)
  line L630 (3.8489, -6.4149) -> (3.0393, -6.4149)
  line L631 (3.9917, -5.9863) -> (4.0393, -5.8435)
  line L632 (4.0393, -5.8435) -> (4.0393, -5.6054)
  line L633 (4.0393, -5.6054) -> (3.9917, -5.5102)
  line L634 (3.9917, -5.5102) -> (3.9441, -5.4625)
  line L635 (3.9441, -5.4625) -> (3.8489, -5.4149)
  line L636 (3.8489, -5.4149) -> (3.7536, -5.4149)
  line L637 (3.7536, -5.4149) -> (3.6584, -5.4625)
  line L638 (3.6584, -5.4625) -> (3.6108, -5.5102)
  line L639 (3.6108, -5.5102) -> (3.5632, -5.6054)
  line L640 (3.5632, -5.6054) -> (3.5155, -5.7959)
  line L641 (3.5155, -5.7959) -> (3.4679, -5.8911)
  line L642 (3.4679, -5.8911) -> (3.4203, -5.9387)
  line L643 (3.4203, -5.9387) -> (3.3251, -5.9863)
  line L644 (3.3251, -5.9863) -> (3.2298, -5.9863)
  line L645 (3.2298, -5.9863) -> (3.1346, -5.9387)
  line L646 (3.1346, -5.9387) -> (3.087, -5.8911)
  line L647 (3.087, -5.8911) -> (3.0393, -5.7959)
  line L648 (3.0393, -5.7959) -> (3.0393, -5.5578)
  line L649 (3.0393, -5.5578) -> (3.087, -5.4149)
  line L650 (3.5155, -4.653) -> (3.5632, -4.5102)
  line L651 (3.5632, -4.5102) -> (3.6108, -4.4625)
  line L652 (3.6108, -4.4625) -> (3.706, -4.4149)
  line L653 (3.706, -4.4149) -> (3.8489, -4.4149)
  line L654 (3.8489, -4.4149) -> (3.9441, -4.4625)
  line L655 (3.9441, -4.4625) -> (3.9917, -4.5102)
  line L656 (3.9917, -4.5102) -> (4.0393, -4.6054)
  line L657 (4.0393, -4.6054) -> (4.0393, -4.9863)
  line L658 (4.0393, -4.9863) -> (3.0393, -4.9863)
  line L659 (3.0393, -4.9863) -> (3.0393, -4.653)
  line L660 (3.0393, -4.653) -> (3.087, -4.5578)
  line L661 (3.087, -4.5578) -> (3.1346, -4.5102)
  line L662 (3.1346, -4.5102) -> (3.2298, -4.4625)
  line L663 (3.2298, -4.4625) -> (3.3251, -4.4625)
  line L664 (3.3251, -4.4625) -> (3.4203, -4.5102)
  line L665 (3.4203, -4.5102) -> (3.4679, -4.5578)
  line L666 (3.4679, -4.5578) -> (3.5155, -4.653)
  line L667 (3.5155, -4.653) -> (3.5155, -4.9863)
  line L668 (4.0393, -3.4625) -> (4.0393, -4.034)
  line L669 (4.0393, -3.7482) -> (3.0393, -3.7482)
  line L670 (3.0393, -3.7482) -> (3.1822, -3.8435)
  line L671 (3.1822, -3.8435) -> (3.2774, -3.9387)
  line L672 (3.2774, -3.9387) -> (3.3251, -4.034)
  line L673 (5.0632, -32.4744) -> (5.5393, -32.4744)
  line L674 (4.5393, -32.8078) -> (5.0632, -32.4744)
  line L675 (5.0632, -32.4744) -> (4.5393, -32.1411)
  line L676 (5.5393, -31.284) -> (5.5393, -31.8554)
  line L677 (5.5393, -31.5697) -> (4.5393, -31.5697)
  line L678 (4.5393, -31.5697) -> (4.6822, -31.6649)
  line L679 (4.6822, -31.6649) -> (4.7774, -31.7602)
  line L680 (4.7774, -31.7602) -> (4.8251, -31.8554)
  line L681 (2.0393, -34.1017) -> (2.0393, -33.4827)
  line L682 (2.0393, -33.4827) -> (2.4203, -33.816)
  line L683 (2.4203, -33.816) -> (2.4203, -33.6731)
  line L684 (2.4203, -33.6731) -> (2.4679, -33.5779)
  line L685 (2.4679, -33.5779) -> (2.5155, -33.5303)
  line L686 (2.5155, -33.5303) -> (2.6108, -33.4827)
  line L687 (2.6108, -33.4827) -> (2.8489, -33.4827)
  line L688 (2.8489, -33.4827) -> (2.9441, -33.5303)
  line L689 (2.9441, -33.5303) -> (2.9917, -33.5779)
  line L690 (2.9917, -33.5779) -> (3.0393, -33.6731)
  line L691 (3.0393, -33.6731) -> (3.0393, -33.9588)
  line L692 (3.0393, -33.9588) -> (2.9917, -34.0541)
  line L693 (2.9917, -34.0541) -> (2.9441, -34.1017)
  line L694 (2.1346, -33.1017) -> (2.087, -33.0541)
  line L695 (2.087, -33.0541) -> (2.0393, -32.9588)
  line L696 (2.0393, -32.9588) -> (2.0393, -32.7208)
  line L697 (2.0393, -32.7208) -> (2.087, -32.6255)
  line L698 (2.087, -32.6255) -> (2.1346, -32.5779)
  line L699 (2.1346, -32.5779) -> (2.2298, -32.5303)
  line L700 (2.2298, -32.5303) -> (2.3251, -32.5303)
  line L701 (2.3251, -32.5303) -> (2.4679, -32.5779)
  line L702 (2.4679, -32.5779) -> (3.0393, -33.1493)
  line L703 (3.0393, -33.1493) -> (3.0393, -32.5303)
  line L704 (2.9441, -32.1017) -> (2.9917, -32.0541)
  line L705 (2.9917, -32.0541) -> (3.0393, -32.1017)
  line L706 (3.0393, -32.1017) -> (2.9917, -32.1493)
  line L707 (2.9917, -32.1493) -> (2.9441, -32.1017)
  line L708 (2.9441, -32.1017) -> (3.0393, -32.1017)
  line L709 (2.0393, -31.7208) -> (2.0393, -31.0541)
  line L710 (2.0393, -31.0541) -> (3.0393, -31.4827)
  line L711 (2.0393, -30.2446) -> (2.0393, -30.435)
  line L712 (2.0393, -30.435) -> (2.087, -30.5303)
  line L713 (2.087, -30.5303) -> (2.1346, -30.5779)
  line L714 (2.1346, -30.5779) -> (2.2774, -30.6731)
  line L715 (2.2774, -30.6731) -> (2.4679, -30.7208)
  line L716 (2.4679, -30.7208) -> (2.8489, -30.7208)
  line L717 (2.8489, -30.7208) -> (2.9441, -30.6731)
  line L718 (2.9441, -30.6731) -> (2.9917, -30.6255)
  line L719 (2.9917, -30.6255) -> (3.0393, -30.5303)
  line L720 (3.0393, -30.5303) -> (3.0393, -30.3398)
  line L721 (3.0393, -30.3398) -> (2.9917, -30.2446)
  line L722 (2.9917, -30.2446) -> (2.9441, -30.1969)
  line L723 (2.9441, -30.1969) -> (2.8489, -30.1493)
  line L724 (2.8489, -30.1493) -> (2.6108, -30.1493)
  line L725 (2.6108, -30.1493) -> (2.5155, -30.1969)
  line L726 (2.5155, -30.1969) -> (2.4679, -30.2446)
  line L727 (2.4679, -30.2446) -> (2.4203, -30.3398)
  line L728 (2.4203, -30.3398) -> (2.4203, -30.5303)
  line L729 (2.4203, -30.5303) -> (2.4679, -30.6255)
  line L730 (2.4679, -30.6255) -> (2.5155, -30.6731)
  line L731 (2.5155, -30.6731) -> (2.6108, -30.7208)
  line L732 (2.4679, -29.5779) -> (2.4203, -29.6731)
  line L733 (2.4203, -29.6731) -> (2.3727, -29.7208)
  line L734 (2.3727, -29.7208) -> (2.2774, -29.7684)
  line L735 (2.2774, -29.7684) -> (2.2298, -29.7684)
  line L736 (2.2298, -29.7684) -> (2.1346, -29.7208)
  line L737 (2.1346, -29.7208) -> (2.087, -29.6731)
  line L738 (2.087, -29.6731) -> (2.0393, -29.5779)
  line L739 (2.0393, -29.5779) -> (2.0393, -29.3874)
  line L740 (2.0393, -29.3874) -> (2.087, -29.2922)
  line L741 (2.087, -29.2922) -> (2.1346, -29.2446)
  line L742 (2.1346, -29.2446) -> (2.2298, -29.1969)
  line L743 (2.2298, -29.1969) -> (2.2774, -29.1969)
  line L744 (2.2774, -29.1969) -> (2.3727, -29.2446)
  line L745 (2.3727, -29.2446) -> (2.4203, -29.2922)
  line L746 (2.4203, -29.2922) -> (2.4679, -29.3874)
  line L747 (2.4679, -29.3874) -> (2.4679, -29.5779)
  line L748 (2.4679, -29.5779) -> (2.5155, -29.6731)
  line L749 (2.5155, -29.6731) -> (2.5632, -29.7208)
  line L750 (2.5632, -29.7208) -> (2.6584, -29.7684)
  line L751 (2.6584, -29.7684) -> (2.8489, -29.7684)
  line L752 (2.8489, -29.7684) -> (2.9441, -29.7208)
  line L753 (2.9441, -29.7208) -> (2.9917, -29.6731)
  line L754 (2.9917, -29.6731) -> (3.0393, -29.5779)
  line L755 (3.0393, -29.5779) -> (3.0393, -29.3874)
  line L756 (3.0393, -29.3874) -> (2.9917, -29.2922)
  line L757 (2.9917, -29.2922) -> (2.9441, -29.2446)
  line L758 (2.9441, -29.2446) -> (2.8489, -29.1969)
  line L759 (2.8489, -29.1969) -> (2.6584, -29.1969)
  line L760 (2.6584, -29.1969) -> (2.5632, -29.2446)
  line L761 (2.5632, -29.2446) -> (2.5155, -29.2922)
  line L762 (2.5155, -29.2922) -> (2.4679, -29.3874)
  line L763 (3.0393, -28.0065) -> (2.0393, -28.0065)
  line L764 (3.0393, -27.435) -> (2.4679, -27.8636)
  line L765 (2.0393, -27.435) -> (2.6108, -28.0065)
  line L766 (3.0393, -27.0065) -> (2.0393, -27.0065)
  line L767 (2.5155, -27.0065) -> (2.5155, -26.435)
  line L768 (3.0393, -26.435) -> (2.0393, -26.435)
  line L769 (2.3727, -26.0541) -> (2.3727, -25.5303)
  line L770 (2.3727, -25.5303) -> (3.0393, -26.0541)
  line L771 (3.0393, -26.0541) -> (3.0393, -25.5303)
  line L772 (55.6536, -19.9293) -> (55.7964, -19.9769)
  line L773 (55.7964, -19.9769) -> (55.844, -20.0245)
  line L774 (55.844, -20.0245) -> (55.8917, -20.1197)
  line L775 (55.8917, -20.1197) -> (55.8917, -20.2626)
  line L776 (55.8917, -20.2626) -> (55.844, -20.3578)
  line L777 (55.844, -20.3578) -> (55.7964, -20.4054)
  line L778 (55.7964, -20.4054) -> (55.7012, -20.4531)
  line L779 (55.7012, -20.4531) -> (55.3202, -20.4531)
  line L780 (55.3202, -20.4531) -> (55.3202, -19.4531)
  line L781 (55.3202, -19.4531) -> (55.6536, -19.4531)
  line L782 (55.6536, -19.4531) -> (55.7488, -19.5007)
  line L783 (55.7488, -19.5007) -> (55.7964, -19.5483)
  line L784 (55.7964, -19.5483) -> (55.844, -19.6435)
  line L785 (55.844, -19.6435) -> (55.844, -19.7388)
  line L786 (55.844, -19.7388) -> (55.7964, -19.834)
  line L787 (55.7964, -19.834) -> (55.7488, -19.8816)
  line L788 (55.7488, -19.8816) -> (55.6536, -19.9293)
  line L789 (55.6536, -19.9293) -> (55.3202, -19.9293)
  line L790 (56.225, -19.4531) -> (56.8917, -19.4531)
  line L791 (56.8917, -19.4531) -> (56.225, -20.4531)
  line L792 (56.225, -20.4531) -> (56.8917, -20.4531)
  line L793 (57.7964, -20.4531) -> (57.225, -20.4531)
  line L794 (57.5107, -20.4531) -> (57.5107, -19.4531)
  line L795 (57.5107, -19.4531) -> (57.4155, -19.5959)
  line L796 (57.4155, -19.5959) -> (57.3202, -19.6912)
  line L797 (57.3202, -19.6912) -> (57.225, -19.7388)
  line L798 (52.9036, -25.2721) -> (53.6655, -25.2721)
  line L799 (53.2845, -25.6531) -> (53.2845, -24.8912)
  line L800 (13.3326, -16.3231) -> (13.3326, -17.1326)
  line L801 (13.3326, -17.1326) -> (13.3802, -17.2278)
  line L802 (13.3802, -17.2278) -> (13.4279, -17.2754)
  line L803 (13.4279, -17.2754) -> (13.5231, -17.3231)
  line L804 (13.5231, -17.3231) -> (13.7136, -17.3231)
  line L805 (13.7136, -17.3231) -> (13.8088, -17.2754)
  line L806 (13.8088, -17.2754) -> (13.8564, -17.2278)
  line L807 (13.8564, -17.2278) -> (13.904, -17.1326)
  line L808 (13.904, -17.1326) -> (13.904, -16.3231)
  line L809 (14.3326, -16.4183) -> (14.3802, -16.3707)
  line L810 (14.3802, -16.3707) -> (14.4755, -16.3231)
  line L811 (14.4755, -16.3231) -> (14.7136, -16.3231)
  line L812 (14.7136, -16.3231) -> (14.8088, -16.3707)
  line L813 (14.8088, -16.3707) -> (14.8564, -16.4183)
  line L814 (14.8564, -16.4183) -> (14.904, -16.5135)
  line L815 (14.904, -16.5135) -> (14.904, -16.6088)
  line L816 (14.904, -16.6088) -> (14.8564, -16.7516)
  line L817 (14.8564, -16.7516) -> (14.285, -17.3231)
  line L818 (14.285, -17.3231) -> (14.904, -17.3231)
  line L819 (10.8326, -29.6031) -> (10.8326, -28.6031)
  line L820 (10.8326, -28.6031) -> (11.0707, -28.6031)
  line L821 (11.0707, -28.6031) -> (11.2136, -28.6507)
  line L822 (11.2136, -28.6507) -> (11.3088, -28.7459)
  line L823 (11.3088, -28.7459) -> (11.3564, -28.8412)
  line L824 (11.3564, -28.8412) -> (11.404, -29.0316)
  line L825 (11.404, -29.0316) -> (11.404, -29.1745)
  line L826 (11.404, -29.1745) -> (11.3564, -29.365)
  line L827 (11.3564, -29.365) -> (11.3088, -29.4602)
  line L828 (11.3088, -29.4602) -> (11.2136, -29.5555)
  line L829 (11.2136, -29.5555) -> (11.0707, -29.6031)
  line L830 (11.0707, -29.6031) -> (10.8326, -29.6031)
  line L831 (11.785, -29.5555) -> (11.9279, -29.6031)
  line L832 (11.9279, -29.6031) -> (12.166, -29.6031)
  line L833 (12.166, -29.6031) -> (12.2612, -29.5555)
  line L834 (12.2612, -29.5555) -> (12.3088, -29.5078)
  line L835 (12.3088, -29.5078) -> (12.3564, -29.4126)
  line L836 (12.3564, -29.4126) -> (12.3564, -29.3174)
  line L837 (12.3564, -29.3174) -> (12.3088, -29.2221)
  line L838 (12.3088, -29.2221) -> (12.2612, -29.1745)
  line L839 (12.2612, -29.1745) -> (12.166, -29.1269)
  line L840 (12.166, -29.1269) -> (11.9755, -29.0793)
  line L841 (11.9755, -29.0793) -> (11.8802, -29.0316)
  line L842 (11.8802, -29.0316) -> (11.8326, -28.984)
  line L843 (11.8326, -28.984) -> (11.785, -28.8888)
  line L844 (11.785, -28.8888) -> (11.785, -28.7935)
  line L845 (11.785, -28.7935) -> (11.8326, -28.6983)
  line L846 (11.8326, -28.6983) -> (11.8802, -28.6507)
  line L847 (11.8802, -28.6507) -> (11.9755, -28.6031)
  line L848 (11.9755, -28.6031) -> (12.2136, -28.6031)
  line L849 (12.2136, -28.6031) -> (12.3564, -28.6507)
  line L850 (13.3088, -29.6031) -> (12.7374, -29.6031)
  line L851 (13.0231, -29.6031) -> (13.0231, -28.6031)
  line L852 (13.0231, -28.6031) -> (12.9279, -28.7459)
  line L853 (12.9279, -28.7459) -> (12.8326, -28.8412)
  line L854 (12.8326, -28.8412) -> (12.7374, -28.8888)
  line L855 (13.6421, -28.6031) -> (14.2612, -28.6031)
  line L856 (14.2612, -28.6031) -> (13.9279, -28.984)
  line L857 (13.9279, -28.984) -> (14.0707, -28.984)
  line L858 (14.0707, -28.984) -> (14.166, -29.0316)
  line L859 (14.166, -29.0316) -> (14.2136, -29.0793)
  line L860 (14.2136, -29.0793) -> (14.2612, -29.1745)
  line L861 (14.2612, -29.1745) -> (14.2612, -29.4126)
  line L862 (14.2612, -29.4126) -> (14.2136, -29.5078)
  line L863 (14.2136, -29.5078) -> (14.166, -29.5555)
  line L864 (14.166, -29.5555) -> (14.0707, -29.6031)
  line L865 (14.0707, -29.6031) -> (13.785, -29.6031)
  line L866 (13.785, -29.6031) -> (13.6898, -29.5555)
  line L867 (13.6898, -29.5555) -> (13.6421, -29.5078)
  line L868 (14.8802, -28.6031) -> (14.9755, -28.6031)
  line L869 (14.9755, -28.6031) -> (15.0707, -28.6507)
  line L870 (15.0707, -28.6507) -> (15.1183, -28.6983)
  line L871 (15.1183, -28.6983) -> (15.166, -28.7935)
  line L872 (15.166, -28.7935) -> (15.2136, -28.984)
  line L873 (15.2136, -28.984) -> (15.2136, -29.2221)
  line L874 (15.2136, -29.2221) -> (15.166, -29.4126)
  line L875 (15.166, -29.4126) -> (15.1183, -29.5078)
  line L876 (15.1183, -29.5078) -> (15.0707, -29.5555)
  line L877 (15.0707, -29.5555) -> (14.9755, -29.6031)
  line L878 (14.9755, -29.6031) -> (14.8802, -29.6031)
  line L879 (14.8802, -29.6031) -> (14.785, -29.5555)
  line L880 (14.785, -29.5555) -> (14.7374, -29.5078)
  line L881 (14.7374, -29.5078) -> (14.6898, -29.4126)
  line L882 (14.6898, -29.4126) -> (14.6421, -29.2221)
  line L883 (14.6421, -29.2221) -> (14.6421, -28.984)
  line L884 (14.6421, -28.984) -> (14.6898, -28.7935)
  line L885 (14.6898, -28.7935) -> (14.7374, -28.6983)
  line L886 (14.7374, -28.6983) -> (14.785, -28.6507)
  line L887 (14.785, -28.6507) -> (14.8802, -28.6031)
  line L888 (15.5945, -28.6983) -> (15.6421, -28.6507)
  line L889 (15.6421, -28.6507) -> (15.7374, -28.6031)
  line L890 (15.7374, -28.6031) -> (15.9755, -28.6031)
  line L891 (15.9755, -28.6031) -> (16.0707, -28.6507)
  line L892 (16.0707, -28.6507) -> (16.1183, -28.6983)
  line L893 (16.1183, -28.6983) -> (16.166, -28.7935)
  line L894 (16.166, -28.7935) -> (16.166, -28.8888)
  line L895 (16.166, -28.8888) -> (16.1183, -29.0316)
  line L896 (16.1183, -29.0316) -> (15.5469, -29.6031)
  line L897 (15.5469, -29.6031) -> (16.166, -29.6031)
  line L898 (16.5945, -29.2221) -> (17.3564, -29.2221)
  line L899 (16.9755, -29.6031) -> (16.9755, -28.8412)
  line L900 (15.2512, -38.6531) -> (15.2512, -39.3674)
  line L901 (15.2512, -39.3674) -> (15.2036, -39.5102)
  line L902 (15.2036, -39.5102) -> (15.1083, -39.6054)
  line L903 (15.1083, -39.6054) -> (14.9655, -39.6531)
  line L904 (14.9655, -39.6531) -> (14.8702, -39.6531)
  line L905 (15.6321, -38.6531) -> (16.2512, -38.6531)
  line L906 (16.2512, -38.6531) -> (15.9179, -39.034)
  line L907 (15.9179, -39.034) -> (16.0607, -39.034)
  line L908 (16.0607, -39.034) -> (16.156, -39.0816)
  line L909 (16.156, -39.0816) -> (16.2036, -39.1293)
  line L910 (16.2036, -39.1293) -> (16.2512, -39.2245)
  line L911 (16.2512, -39.2245) -> (16.2512, -39.4626)
  line L912 (16.2512, -39.4626) -> (16.2036, -39.5578)
  line L913 (16.2036, -39.5578) -> (16.156, -39.6054)
  line L914 (16.156, -39.6054) -> (16.0607, -39.6531)
  line L915 (16.0607, -39.6531) -> (15.775, -39.6531)
  line L916 (15.775, -39.6531) -> (15.6798, -39.6054)